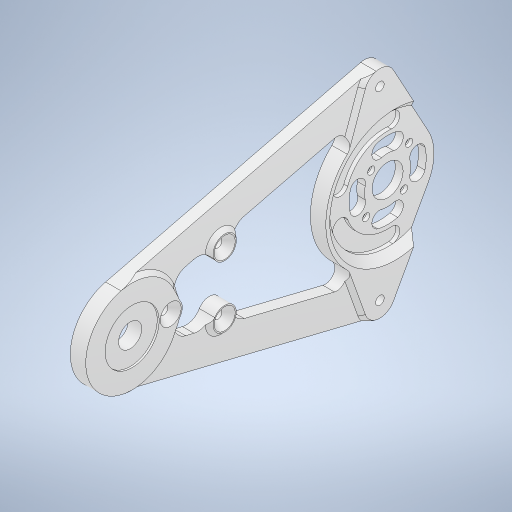
# Autodesk Inventor part: Upright - Motor
Saved by Autodesk Inventor 2023.2 (Build 272271000, 271)
## iProperties
Created: 2023-07-17
Part Number: Upright - Motor
Material: Aluminum 6061
Document SubType Name: Modeling
Designer: Nathan Cai
Mass: 70.1116 g
Surface Area: 173.553 cm^2
Volume: 25.9672 cm^3
Density: 2.7 g/cm^3
Appearance: Aluminum - Flat
C2C: 4.263 in
Bore: 0.375 in
S_Offset: 1.500 in
FrontOD: 1.500 in
Leg_Y_Back: 0.500 in
Leg_X_Back: 1.500 in
Leg_X_Front: 0.625 in
M2S: 0.250 in
Author: Nathan Cai
Autodesk Inventor part; units mm, degrees
ref_plane "YZ Plane" through (0, 0, 0) normal (1, 0, 0) x (0, 1, 0)
ref_plane "XZ Plane" through (0, 0, 0) normal (0, 1, 0) x (-1, 0, 0)
ref_plane "XY Plane" through (0, 0, 0) normal (0, 0, 1) x (1, 0, 0)
sketch "Sketch1" plane through (0, 0, 0) normal (1, 0, 0) x (0, 1, 0)
  circle A0 centre (0, 0) radius 19.05
  circle A1 centre (0, 0) radius 6.35
  circle A2 centre (0, 0) radius 28.575
  line L0 (0, 0) -> (0, 108.2802) construction
  circle A3 centre (0, 108.2802) radius 76.2 construction
  circle A4 centre (0, 108.2802) radius 4.7625
  line L1 (0, 6.35) -> (0, -38.1) construction
  line L2 (0, 6.35) -> (38.1, 6.35) construction
  circle A5 centre (38.1, 6.35) radius 1.7526
  circle A6 centre (38.1, 6.35) radius 6.35
  circle A7 centre (0, 108.2802) radius 15.875 construction
  circle A8 centre (0, 108.2802) radius 19.05
  line L3 (18.5007, 112.8219) -> (44.2669, 7.8639)
  line L4 (10.4489, 92.3515) -> (31.9331, 4.8361)
  line L5 (41.1454, 0.7779) -> (9.1361, -16.7163)
  arc A9 (20.6423, 19.7592) -> (27.3636, 23.4497) centre (23.5093, 22.5035) ccw
  circle A10 centre (-38.1, 6.35) radius 1.7526
  circle A11 centre (-38.1, 6.35) radius 6.35
  line L6 (-18.5007, 112.8219) -> (-44.2669, 7.8639)
  line L7 (-10.4489, 92.3515) -> (-31.9331, 4.8361)
  line L8 (-41.1454, 0.7779) -> (-9.1361, -16.7163)
  arc A12 (-27.3636, 23.4497) -> (-20.6423, 19.7592) centre (-23.5093, 22.5035) ccw
  circle A13 centre (12.7, 70.1802) radius 1.7526
  circle A14 centre (12.7, 70.1802) radius 4.7625
  circle A15 centre (-12.7, 70.1802) radius 1.7526
  circle A16 centre (-12.7, 70.1802) radius 4.7625
  circle A17 centre (0, 108.2802) radius 9.525 construction
  circle A18 centre (0, 92.4052) radius 1.7526
  circle A19 centre (0, 92.4052) radius 4.7625
  point P0 (-18.5007, 112.8219)
  point P1 (-9.1361, -16.7163)
  point P2 (-16.5723, 67.4078)
  point P3 (-14.8483, 74.4306)
  point P4 (-10.4489, 92.3515)
  point P5 (14.8483, 74.4306)
  point P6 (16.5723, 67.4078)
  point P7 (3.8683, 89.6271)
  point P8 (-3.8683, 89.6271)
  dimension "d0" = 38.1
  dimension "d2" = 57.15
  dimension "d11" = 31.75
  dimension "d1" = 12.7
  dimension "d3" = 152.4
  dimension "C2C" = 108.2802
  dimension "Bore" = 9.525
  dimension "d6" = 44.45
  dimension "M2S" = 6.35
  dimension "S_Offset" = 38.1
  dimension "d9" = 3.5052
  dimension "d10" = 12.7
  dimension "FrontOD" = 38.1
  dimension "d13" = 7.9375
  dimension "d17" = 3.5052
  dimension "d18" = 9.525
  dimension "Leg_Y_Back" = 12.7
  dimension "Leg_X_Back" = 38.1
  dimension "d21" = 19.05
  dimension "d22" = 3.5052
  dimension "d51" = 9.525
  dimension "Leg_X_Front" = 15.875
  constraints: 18 end point, 17 centre point, 14 coincident, 13 symmetric about line, 12 point on circle, 5 point on line, 5 tangent, 1 parallel, 1 perpendicular, 1 vertical, 1 vertical alignment, 15 other
  measures "d1" diameter of A1
  measures "d3" diameter of A3
  measures "C2C" distance of L0.start L0.end
  measures "Bore" diameter of A4
  measures "d6" distance of L1.start L1.end
  measures "M2S" distance of point (0, 0) L1.start
  measures "S_Offset" distance of L1.start L2.end
  measures "d9" diameter of A5
  measures "d10" diameter of A6
  measures "FrontOD" diameter of A8
  measures "d13" diameter of A9
  measures "d17" diameter of A13
  measures "d18" diameter of A14
  measures "Leg_Y_Back" distance from line of L0 A14.centre
  measures "Leg_X_Back" vertical distance of A4.centre A14.centre
  measures "d21" diameter of A17
  measures "d22" diameter of A18
  measures "d51" diameter of A19
  measures "Leg_X_Front" distance of A4.centre A18.centre
extrude "Extrusion1" add sketch "Sketch1" along normal blind 6.35 contours A0 | A0 L8 A2 L5 | L8 A11 L7 A12 A2 | A2 A9 L4 A6 L5 | A11 | A6 | L7 A11 L6 A8 A16 | L4 A14 A8 L3 A6 | A16 L7 | L7 A16 | A8 A19 | A14 L4 | L4 A14 | A19 A8 | A8 A19 picked at (-25.1284, -2.4933)
fillet "Fillet1" radius 6.35 8 edges at (3.175, 10.4489, 92.3515) (3.175, 14.8483, 74.4306) (3.175, 16.5723, 67.4078) (3.175, -10.4489, 92.3515) (3.175, -14.8483, 74.4306) (3.175, -16.5723, 67.4078) (3.175, 3.8683, 89.6271) (3.175, -3.8683, 89.6271)
sketch "Sketch3" plane through (6.35, 0, 0) normal (1, 0, 0) x (0, 0, -1)
  circle A0 centre (0, 0) radius 23.8125
  dimension "d30" = 47.625
  constraints: 1 centre point, 1 coincident
  measures "d30" diameter of A0
extrude "Extrusion3" cut sketch "Sketch3" against normal blind 3.175
sketch "Sketch4" plane through (6.35, 0, 0) normal (1, 0, 0) x (0, 0, -1)
  circle A0 centre (-108.2802, 0) radius 4.7625 projected
  circle A1 centre (-108.2802, 0) radius 11.1125
  point P0 (0, 0)
  dimension "d36" = 22.225
  constraints: 1 centre point, 1 coincident
  measures "d36" diameter of A1
extrude "Extrusion4" cut sketch "Sketch4" against normal blind 0.7937
chamfer "Chamfer7" distance 3.175 angle 45 1 edges at (6.35, 0, 23.8125)
sketch "Sketch7" plane through (6.35, 0, 0) normal (1, 0, 0) x (0, 0, -1)
  circle A0 centre (-108.2802, 0) radius 4.7625 projected
  line L0 (0, 0) -> (-108.2802, 0) construction
  circle A1 centre (-6.35, -38.1) radius 1.7526 projected
  arc A2 (-7.8639, -44.2669) -> (-0.7779, -41.1454) centre (-6.35, -38.1) ccw projected
  circle A3 centre (-6.35, -38.1) radius 6.35
  line L1 (-12.3316, -40.2315) -> (-18.765, -22.1772)
  arc A4 (-23.4497, -27.3636) -> (-19.7592, -20.6423) centre (-22.5035, -23.5093) ccw projected
  circle A5 centre (-70.1802, -12.7) radius 1.7526 projected
  arc A6 (-65.4252, -12.433) -> (-74.271, -10.2614) centre (-70.1802, -12.7) ccw projected
  circle A7 centre (-70.1802, -12.7) radius 4.7625
  circle A8 centre (-92.4052, 0) radius 1.7526 projected
  arc A9 (-88.4433, -2.6428) -> (-84.6746, -12.3335) centre (-83.1607, -6.1666) ccw projected
  circle A10 centre (-92.4052, 0) radius 4.7625
  line L2 (-88.1189, -2.0759) -> (-91.1352, -8.3037)
  arc A11 (-112.8219, 18.5007) -> (-112.8219, -18.5007) centre (-108.2802, 0) ccw projected
  arc A12 (-88.4433, -2.6428) -> (-88.4433, 2.6428) centre (-92.4052, 0) ccw projected
  line L3 (-112.8219, -18.5007) -> (-7.8639, -44.2669) projected
  circle A13 centre (-108.2802, 0) radius 19.05
  arc A14 (7.5486, 25.9103) -> (7.5486, -25.9103) centre (0, 0) ccw projected
  line L4 (7.5486, 25.9103) -> (-0.7779, 41.1454) projected
  arc A15 (-0.7779, 41.1454) -> (-7.8639, 44.2669) centre (-6.35, 38.1) ccw projected
  line L5 (-7.8639, 44.2669) -> (-112.8219, 18.5007) projected
  arc A16 (-112.8219, 18.5007) -> (-112.8219, -18.5007) centre (-108.2802, 0) ccw projected
  line L6 (-112.8219, -18.5007) -> (-7.8639, -44.2669) projected
  arc A17 (-7.8639, -44.2669) -> (-0.7779, -41.1454) centre (-6.35, -38.1) ccw projected
  line L7 (-0.7779, -41.1454) -> (7.5486, -25.9103) projected
  circle A18 centre (-108.2802, 0) radius 11.1125 projected
  circle A19 centre (-6.35, 38.1) radius 1.7526 projected
  circle A20 centre (-70.1802, 12.7) radius 1.7526 projected
  circle A21 centre (-6.35, -38.1) radius 1.7526 projected
  circle A22 centre (-70.1802, -12.7) radius 1.7526 projected
  circle A23 centre (-92.4052, 0) radius 1.7526 projected
  arc A24 (-84.6746, 12.3335) -> (-88.4433, 2.6428) centre (-83.1607, 6.1666) ccw projected
  line L8 (-84.6746, 12.3335) -> (-81.2393, 13.1768) projected
  arc A25 (-74.271, 10.2614) -> (-81.2393, 13.1768) centre (-79.7254, 7.0099) ccw projected
  arc A26 (-74.271, 10.2614) -> (-65.4252, 12.433) centre (-70.1802, 12.7) ccw projected
  arc A27 (-60.5991, 18.2438) -> (-65.4252, 12.433) centre (-59.0852, 12.0769) ccw projected
  line L9 (-60.5991, 18.2438) -> (-23.4497, 27.3636) projected
  arc A28 (-19.7592, 20.6423) -> (-23.4497, 27.3636) centre (-22.5035, 23.5093) ccw projected
  arc A29 (-19.7592, 20.6423) -> (-19.7592, -20.6423) centre (0, 0) ccw projected
  arc A30 (-23.4497, -27.3636) -> (-19.7592, -20.6423) centre (-22.5035, -23.5093) ccw projected
  line L10 (-23.4497, -27.3636) -> (-60.5991, -18.2438) projected
  arc A31 (-65.4252, -12.433) -> (-60.5991, -18.2438) centre (-59.0852, -12.0769) ccw projected
  arc A32 (-65.4252, -12.433) -> (-74.271, -10.2614) centre (-70.1802, -12.7) ccw projected
  arc A33 (-81.2393, -13.1768) -> (-74.271, -10.2614) centre (-79.7254, -7.0099) ccw projected
  line L11 (-81.2393, -13.1768) -> (-84.6746, -12.3335) projected
  arc A34 (-88.4433, -2.6428) -> (-84.6746, -12.3335) centre (-83.1607, -6.1666) ccw projected
  arc A35 (-88.4433, -2.6428) -> (-88.4433, 2.6428) centre (-92.4052, 0) ccw projected
  circle A36 centre (-6.35, 38.1) radius 6.35
  line L12 (-12.3316, 40.2315) -> (-18.765, 22.1772)
  circle A37 centre (-70.1802, 12.7) radius 4.7625
  line L13 (-88.1189, 2.0759) -> (-91.1352, 8.3037)
  point P0 (-74.271, 10.2614)
  point P1 (-7.8639, 44.2669)
  point P2 (-112.8219, 18.5007)
  point P3 (-89.2817, 4.4768)
  point P4 (-74.271, -10.2614)
  point P5 (-84.6746, -12.3335)
  point P6 (-89.2817, -4.4768)
  constraints: 10 end point, 7 point on circle, 6 symmetric about line, 4 centre point, 4 coincident, 4 tangent, 1 horizontal, 8 other
extrude "Extrusion8" cut sketch "Sketch7" against normal blind 1.5875 contours L3 A13 L2 A9 L11 A33 A7 A31 L10 A4 L1 A3 | L5 A36 L12 A28 L9 A27 A37 A25 L8 A24 L13 A13
chamfer "Chamfer8" distance 1.5875 angle 45 10 edges at (4.7625, 17.2394, 100.1743) (4.7625, 6.3912, 90.2089) (4.7625, -6.3912, 90.2089) (4.7625, -17.2394, 100.1743) (4.7625, 17.3252, 71.3156) (4.7625, -17.3252, 71.3156) (4.7625, 31.2043, 15.5483) (4.7625, 42.8123, 10.6064) (4.7625, -31.2043, 15.5483) (4.7625, -42.8123, 10.6064)
sketch "Sketch5" plane through (3.175, 0, 0) normal (-1, 0, 0) x (0, 0, 1)
  circle A0 centre (0, 0) radius 8 construction
  circle A1 centre (0, 0) radius 9.5 construction
  circle A2 centre (0, 0) radius 12.5 construction
  line L0 (0, 0) -> (0, 12.5) construction
  line L1 (0, 0) -> (8.8388, 8.8388) construction
  line L2 (0, 0) -> (-8.8388, 8.8388) construction
  circle A3 centre (6.7175, 6.7175) radius 1.5
  circle A4 centre (-8.8388, 8.8388) radius 1.5
  circle A5 centre (8.8388, -8.8388) radius 1.5
  circle A6 centre (-6.7175, -6.7175) radius 1.5
  circle A7 centre (0, 0) radius 12.7 construction
  arc A8 (3.287, 12.2673) -> (-3.287, 12.2673) centre (0, 0) ccw construction
  arc A9 (4.1088, 15.3341) -> (-4.1088, 15.3341) centre (0, 0) ccw
  arc A10 (2.4653, 9.2004) -> (-2.4653, 9.2004) centre (0, 0) ccw
  arc A11 (2.4653, 9.2004) -> (4.1088, 15.3341) centre (3.287, 12.2673) ccw
  arc A12 (-4.1088, 15.3341) -> (-2.4653, 9.2004) centre (-3.287, 12.2673) ccw
  line L3 (-3.287, 12.2673) -> (0, 0) construction
  line L4 (0, 0) -> (3.287, 12.2673) construction
  arc A13 (-9.2004, 2.4653) -> (-9.2004, -2.4653) centre (0, 0) ccw
  arc A14 (-9.2004, 2.4653) -> (-15.3341, 4.1088) centre (-12.2673, 3.287) ccw
  arc A15 (-15.3341, -4.1088) -> (-9.2004, -2.4653) centre (-12.2673, -3.287) ccw
  arc A16 (-15.3341, 4.1088) -> (-15.3341, -4.1088) centre (0, 0) ccw
  arc A17 (-12.2673, 3.287) -> (-12.2673, -3.287) centre (0, 0) ccw construction
  arc A18 (-2.4653, -9.2004) -> (2.4653, -9.2004) centre (0, 0) ccw
  arc A19 (-2.4653, -9.2004) -> (-4.1088, -15.3341) centre (-3.287, -12.2673) ccw
  arc A20 (4.1088, -15.3341) -> (2.4653, -9.2004) centre (3.287, -12.2673) ccw
  arc A21 (-4.1088, -15.3341) -> (4.1088, -15.3341) centre (0, 0) ccw
  arc A22 (-3.287, -12.2673) -> (3.287, -12.2673) centre (0, 0) ccw construction
  arc A23 (9.2004, -2.4653) -> (9.2004, 2.4653) centre (0, 0) ccw
  arc A24 (9.2004, -2.4653) -> (15.3341, -4.1088) centre (12.2673, -3.287) ccw
  arc A25 (15.3341, 4.1088) -> (9.2004, 2.4653) centre (12.2673, 3.287) ccw
  arc A26 (15.3341, -4.1088) -> (15.3341, 4.1088) centre (0, 0) ccw
  arc A27 (12.2673, -3.287) -> (12.2673, 3.287) centre (0, 0) ccw construction
  arc A28 (19.3929, 7.0584) -> (-1.7987, 20.559) centre (0, 0) ccw construction
  arc A29 (22.3764, 8.1444) -> (-2.0754, 23.7219) centre (0, 0) ccw
  arc A30 (16.4094, 5.9725) -> (-1.522, 17.396) centre (0, 0) ccw
  arc A31 (16.4094, 5.9725) -> (22.3764, 8.1444) centre (19.3929, 7.0584) ccw
  arc A32 (-2.0754, 23.7219) -> (-1.522, 17.396) centre (-1.7987, 20.559) ccw
  line L5 (0, 0) -> (-1.7987, 20.559) construction
  line L6 (0, 0) -> (19.3929, 7.0584) construction
  line L7 (0, 0) -> (6.35, 0) construction
  circle A33 centre (0, 0) radius 6.35 projected
  arc A34 (-2.0754, -23.7219) -> (22.3764, -8.1444) centre (0, 0) ccw
  arc A35 (-1.522, -17.396) -> (16.4094, -5.9725) centre (0, 0) ccw
  arc A36 (22.3764, -8.1444) -> (16.4094, -5.9725) centre (19.3929, -7.0584) ccw
  arc A37 (-1.522, -17.396) -> (-2.0754, -23.7219) centre (-1.7987, -20.559) ccw
  circle A38 centre (0, 0) radius 16 construction
  point P0 (-12.5, 0)
  point P1 (0, -12.5)
  point P2 (12.5, 0)
  dimension "d57" = 19
  dimension "d66" = 25.4
  dimension "d56" = 16
  dimension "d58" = 25
  dimension "d59" = 45
  dimension "d60" = 3
  dimension "d61" = 3
  dimension "d64" = 360
  dimension "d67" = 6.35
  dimension "d68" = 30
  dimension "d69" = 30
  dimension "d72" = 360
  dimension "d74" = 20.6375
  dimension "d75" = 6.35
  dimension "d76" = 5
  dimension "d77" = 70
  dimension "d87" = 32
  constraints: 61 point on circle, 36 centre point, 16 end point, 8 coincident, 8 tangent, 6 symmetric about line, 1 horizontal, 1 horizontal alignment, 1 perpendicular, 1 point on line, 1 vertical, 74 other
  measures "d56" diameter of A0
  measures "d58" diameter of A2
  measures "d59" angle of L0 L1
  measures "d60" diameter of A3
  measures "d61" diameter of A4
  measures "d67" diameter of A12
  measures "d68" angle of L2 L3
  measures "d69" angle of L1 L4
  measures "d74" radius of A28
  measures "d75" diameter of A31
  measures "d76" angle of L0 L5
  measures "d77" angle of L0 L6
  measures "d87" diameter of A38
extrude "Extrusion5" cut sketch "Sketch5" along normal blind 1.5875 contours A31 A30 A32 A29 | A37 A35 A36 A34
extrude "Extrusion6" cut sketch "Sketch5" along normal through all contours A3 | A4 | A5 | A6 | A11 A10 A12 A9 | A13 A15 A16 A14 | A18 A20 A21 A19 | A23 A25 A26 A24
chamfer "Chamfer5" distance 2.54 angle 49 3 edges at (6.35, -14.4526, 70.1802) (6.35, 10.9474, 70.1802) (6.35, -1.7526, 92.4052) measured on face at (6.35, 10.4474, 70.1802) measured on face at (6.35, -2.2526, 92.4052) measured on face at (6.35, -14.9526, 70.1802)
chamfer "Chamfer6" distance 1.75 angle 45 4 edges at (0, -8.8388, 7.3388) (0, -6.7175, -8.2175) (0, 8.8388, -10.3388) (0, 6.7175, 5.2175)
body "Solid1"
